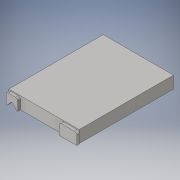
# Autodesk Inventor part: tail stock
Saved by Autodesk Inventor 2016 (Build 200138000, 138)
## iProperties
Created: 2017-02-14
Part Number: tail stock
Material: Generic
Document SubType Name: Modeling
Designer: m207653
Density: 1 g/cm^3
Appearance: Default
Author: m207653
Autodesk Inventor part; units mm, degrees
ref_plane "YZ Plane" through (0, 0, 0) normal (1, 0, 0) x (0, 1, 0)
ref_plane "XZ Plane" through (0, 0, 0) normal (0, 1, 0) x (-1, 0, 0)
ref_plane "XY Plane" through (0, 0, 0) normal (0, 0, 1) x (1, 0, 0)
sketch "Sketch1" plane through (0, 0, 0) normal (0, 1, 0) x (-1, 0, 0)
  line L0 (-14.8781, 49.9341) -> (-14.8781, 23.9341)
  line L1 (-14.8781, 23.9341) -> (-165.8781, 23.9341)
  line L2 (-165.8781, 23.9341) -> (-165.8781, 49.9341)
  line L3 (-165.8781, 49.9341) -> (-14.8781, 49.9341)
  point P0 (0, 0)
  dimension "d19" = 26
  dimension "d20" = 151
  constraints: 8 end point, 3 perpendicular, 1 vertical
  measures "d19" distance of L0.start L0.end
  measures "d20" distance of L0.end L1.end
extrude "Extrusion1" add sketch "Sketch1" along normal blind 203
sketch "Sketch2" plane through (0, 0, 0) normal (0, -1, 0) x (1, 0, 0)
  line L0 (14.8781, 23.9341) -> (14.8781, 49.9341) projected
  line L1 (14.8781, 49.9341) -> (14.8781, 23.9341)
  line L2 (14.8781, 49.9341) -> (39.8781, 49.9341)
  line L3 (14.8781, 49.9341) -> (165.8781, 49.9341) projected
  line L4 (39.8781, 49.9341) -> (39.8781, 23.9341)
  line L5 (165.8781, 23.9341) -> (14.8781, 23.9341) projected
  line L6 (14.8781, 23.9341) -> (39.8781, 23.9341)
  line L7 (27.3781, 49.9341) -> (27.3781, 33.9341)
  line L8 (25.4781, 33.9341) -> (38.7147, 33.9341) construction
  line L9 (29.4781, 36.9341) -> (43.9589, 36.9341) construction
  line L10 (27.3781, 33.9341) -> (29.624, 33.9341)
  line L11 (29.624, 33.9341) -> (25.624, 33.9341)
  line L12 (25.624, 33.9341) -> (17.233, 23.9341)
  line L13 (25.624, 33.9341) -> (51.2693, 33.9341) construction
  line L14 (29.624, 33.9341) -> (38.015, 23.9341)
  line L15 (29.624, 33.9341) -> (59.3837, 33.9341) construction
  point P0 (0, 0)
  dimension "d23" = 25
  dimension "d29" = 4
  dimension "d30" = 130
  dimension "d31" = 50
  dimension "d32" = 10
  constraints: 26 end point, 9 point on line, 4 horizontal, 2 collinear, 1 perpendicular
  measures "d23" distance of L0.end L2.end
  measures "d29" distance of L10.end L11.end
  measures "d30" angle of L12 L13
  measures "d31" angle of L14 L15
  measures "d32" vertical distance of L0.start L11.end
extrude "Extrusion2" cut sketch "Sketch2" against normal blind 215 contours L12 L11 L10 L14 L5
sketch "Sketch3" plane through (0, 0, 0) normal (0, -1, 0) x (1, 0, 0)
  line L0 (14.8781, 23.9341) -> (17.233, 23.9341) projected
  line L1 (14.8781, 49.9341) -> (14.8781, 23.9341) projected
  line L2 (14.8781, 23.9341) -> (14.8781, 49.9341)
  line L3 (14.8781, 49.9341) -> (39.8781, 49.9341)
  line L4 (165.8781, 49.9341) -> (14.8781, 49.9341) projected
  line L5 (39.8781, 49.9341) -> (39.8781, 23.9341)
  line L6 (38.015, 23.9341) -> (165.8781, 23.9341) projected
  line L7 (14.8781, 23.9341) -> (17.233, 23.9341)
  line L8 (17.233, 23.9341) -> (25.624, 33.9341) projected
  line L9 (25.624, 33.9341) -> (17.233, 23.9341)
  line L10 (17.233, 23.9341) -> (25.624, 33.9341)
  line L11 (25.624, 33.9341) -> (29.624, 33.9341) projected
  line L12 (29.624, 33.9341) -> (38.015, 23.9341) projected
  line L13 (29.624, 33.9341) -> (38.015, 23.9341)
  line L14 (38.015, 23.9341) -> (39.8781, 23.9341)
  point P0 (0, 0)
  dimension "d35" = 25
  constraints: 16 end point, 3 collinear, 2 point on line, 1 horizontal, 1 perpendicular, 1 vertical
  measures "d35" distance of L1.start L3.end
extrude "Extrusion3" add sketch "Sketch3" along normal blind 6
sketch "Sketch4" plane through (14.8781, 203, 49.9341) normal (0, 0, 1) x (1, 0, 0)
  line L0 (0, -209) -> (0, -203)
  line L1 (2.3549, 0) -> (2.3549, -209) projected
  line L2 (151, -203) -> (25, -203) projected
  line L3 (0, -203) -> (25, -203)
  line L4 (25, -209) -> (0, -209) projected
  line L5 (25, -203) -> (25, -209)
  line L6 (25, -209) -> (0, -209)
  line L7 (0, -209) -> (0, -203)
  point P0 (-14.8781, -203)
  constraints: 10 end point, 3 perpendicular, 1 collinear, 1 parallel
extrude "Extrusion4" cut sketch "Sketch4" against normal blind 2
sketch "Sketch5" plane through (0, 0, 0) normal (0, -1, 0) x (1, 0, 0)
  line L0 (165.8781, 23.9341) -> (38.015, 23.9341) projected
  line L1 (165.8781, 23.9341) -> (165.8781, 47.9341)
  line L2 (165.8781, 49.9341) -> (165.8781, 23.9341) projected
  line L3 (39.8781, 47.9341) -> (14.8781, 47.9341) projected
  line L4 (165.8781, 47.9341) -> (128.8781, 47.9341)
  line L5 (128.8781, 47.9341) -> (128.8781, 23.9341)
  line L6 (165.8781, 23.9341) -> (128.8781, 23.9341)
  point P0 (0, 0)
  dimension "d40" = 37
  constraints: 8 end point, 3 perpendicular, 2 point on line, 1 collinear
  measures "d40" distance of L1.end L4.end
extrude "Extrusion5" add sketch "Sketch5" along normal blind 6
sketch "Sketch6" plane through (165.8781, 0, 49.9341) normal (1, 0, 0) x (0, 0, -1)
  line L0 (26, -6) -> (2, -6) projected
  line L1 (2, 0) -> (2, -6) projected
  line L2 (2, -6) -> (2, 0)
  line L3 (2, 0) -> (26, 0) projected
  line L4 (2, 0) -> (26, 0)
  line L5 (26, 0) -> (26, -6) projected
  line L6 (26, 0) -> (26, -6)
  line L7 (26, -6) -> (2, -6)
  line L8 (2, -6) -> (2, 0)
  point P0 (49.9341, 0)
  constraints: 10 end point, 4 collinear, 1 perpendicular
extrude "Extrusion6" add sketch "Sketch6" along normal blind 1
fillet "Fillet1" radius 5 2 edges at (166.8781, -3, 47.9341) (128.8781, -3, 47.9341)
fillet "Fillet2" radius 5 2 edges at (39.8781, -3, 47.9341) (14.8781, -3, 47.9341)
body "Solid1"
